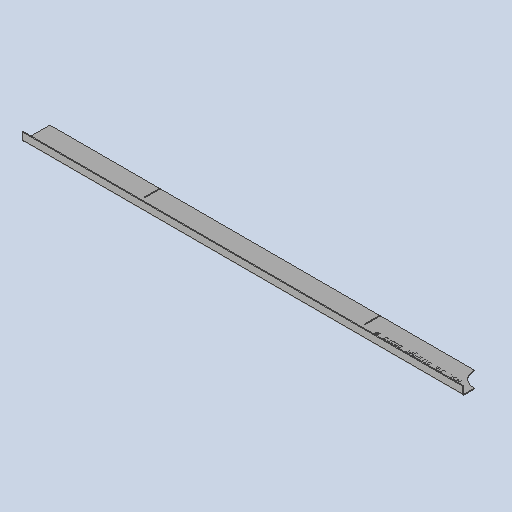
# Autodesk Inventor part: MSC 316 stringer board #
Saved by Autodesk Inventor 2025 (Build 290162010, 162A)
## iProperties
Created: 2024-04-28
Part Number: MSC 316 stringer board #
Material: Stainless Steel
Document SubType Name: Sheet Metal
Designer: pokla
Density: 8 g/cm^3
Sheet Metal Rule: AISI304 2mm Die16
Appearance: Default
Flat Pattern Width: 98 cm
Flat Pattern Length: 7.8202 cm
Flat Pattern Area: 766.38 cm^2
Sheet Metal Width: 980,000 mm
Sheet Metal Length: 78,202 mm
Sheet Metal Area: 76637,951 mm^2
Stock Number: МОО 316 стрингер борт #
Mass: 1211.55 g
Surface Area: 1559.11 cm^2
Volume: 151.444 cm^3
Author: admin
Autodesk Inventor part; units mm, degrees
ref_plane "YZ Plane" through (0, 0, 0) normal (1, 0, 0) x (0, 1, 0)
ref_plane "XZ Plane" through (0, 0, 0) normal (0, 1, 0) x (-1, 0, 0)
ref_plane "XY Plane" through (0, 0, 0) normal (0, 0, 1) x (1, 0, 0)
sketch "Sketch1" plane through (0, 0, 0) normal (0, 0, 1) x (1, 0, 0)
  line L0 (-490, 62) -> (490, 62)
  line L1 (490, 62) -> (490, 0)
  line L2 (490, 0) -> (-490, 0)
  line L3 (-490, 0) -> (-490, 62)
  point P0 (0, 0)
  point P1 (0, 0)
  dimension "d0" = 980
  dimension "d1" = 62
  measures "d0" distance of L1.end L2.end
  measures "d1" distance of L0.end L1.end
extrude "Plate1" add sketch "Sketch1" along normal blind 2
sketch "Sketch2" plane through (490, 2, 0) normal (0, -1, 0) x (1, 0, 0)
  line L0 (-980, 0) -> (0, 0)
  line L1 (0, 0) -> (0, 20)
  line L2 (0, 20) -> (-980, 20)
  line L3 (-980, 20) -> (-980, 0)
  constraints: 6 end point, 1 horizontal, 1 perpendicular, 1 vertical
edge flange "Flange1" height 20 angle 90 thickness 2 bend radius 2.75 thickness toward (0, -1, 0) relief round relief width 2 relief depth 1 edges at (0, 0, 2) wall of the first edge with corners at (-490, 2, 0) (490, 2, 0) (490, 2, 20) (-490, 2, 20)
bend "Bend1"
corner "Corner1"
sketch "Sketch5" plane through (0, 0, 0) normal (0, 0, -1) x (-1, 0, 0)
  line L0 (490, 62) -> (-490, 62) projected
  line L1 (490, 0) -> (-490, 0) projected
  circle A0 centre (0, 62) radius 35
  line L2 (243.95, 62) -> (246.05, 62)
  line L3 (246.05, 62) -> (246.05, 29)
  line L4 (246.05, 29) -> (243.95, 29)
  line L5 (243.95, 29) -> (243.95, 62)
  line L6 (-243.95, 62) -> (-246.05, 62)
  line L7 (-246.05, 62) -> (-246.05, 29)
  line L8 (-246.05, 29) -> (-243.95, 29)
  line L9 (-243.95, 29) -> (-243.95, 62)
  line L10 (0, 62) -> (0, 0) construction
  circle A1 centre (-490, 62) radius 35
  circle A2 centre (490, 62) radius 35
  point P0 (245, 29)
  point P1 (-245, 29)
  point P2 (0, 62)
  point P3 (-35, 62)
  point P4 (35, 62)
  dimension "d39" = 70
  dimension "d40" = 2.1
  dimension "d41" = 490
  dimension "d44" = 29
  dimension "d45" = 33
  constraints: 18 end point, 4 midpoint, 4 parallel, 3 centre point, 3 coincident, 2 collinear, 2 equal radius, 2 horizontal, 2 perpendicular, 1 vertical alignment, 1 other
  measures "d39" diameter of A0
  measures "d40" distance of L8.start L9.start
  measures "d41" distance of point (245, 29) point (-245, 29)
  measures "d44" distance between parallel lines of L1 L8
  measures "d45" distance between parallel lines of L0 L8
extrude "Extrusion4" cut sketch "Sketch5" along normal through all both and the other way through all contours L3 L4 L5 L0 | L9 L8 L7 L0 | A1
sketch "Sketch9" plane through (0, 0, 2) normal (0, 0, 1) x (1, 0, 0)
  line L0 (462.3716, 29.596) -> (462.3716, 17.596) construction
  line L1 (462.3716, 17.596) -> (262.3716, 17.596) construction
  line L2 (262.3716, 17.596) -> (262.3716, 29.596) construction
  line L3 (262.3716, 29.596) -> (462.3716, 29.596) construction
  point P0 (0, 0)
  point P1 (490, 62)
  dimension "d48" = 200
  dimension "d49" = 12
  constraints: 1 horizontal, 2 other
  measures "d48" distance of L0.end L1.end
  measures "d49" distance of L1.end L2.end
mark "Mark3"
equation "\"d1\" = БОРТ_стрингер_3_высота"
equation "\"d2\" = Thickness"
equation "\"d3\" = BendReliefWidth"
equation "\"d4\" = BendReliefDepth"
equation "\"d5\" = MinimumRemnant"
equation "\"d6\" = TransitionRadius"
equation "\"d9\" = BendRadius"
equation "\"d10\" = CornerReliefSize"
equation "\"d11\" = GapSize"
equation "\"d12\" = JacobiRadiusSize"
equation "\"BendReliefWidth\" = Thickness"
equation "\"BendReliefDepth\" = 0.5 * Thickness"
equation "\"CornerReliefSize\" = 4 * Thickness"
equation "\"MinimumRemnant\" = 2 * Thickness"
equation "\"TransitionRadius\" = BendRadius"
equation "\"JacobiRadiusSize\" = BendRadius"
equation "\"GapSize\" = Thickness"
equation "\"БОРТ_стрингер_3_высота\" = 62"
equation "\"Thickness\" = 2"
equation "\"BendRadius\" = 2.75"
body "Solid1"
